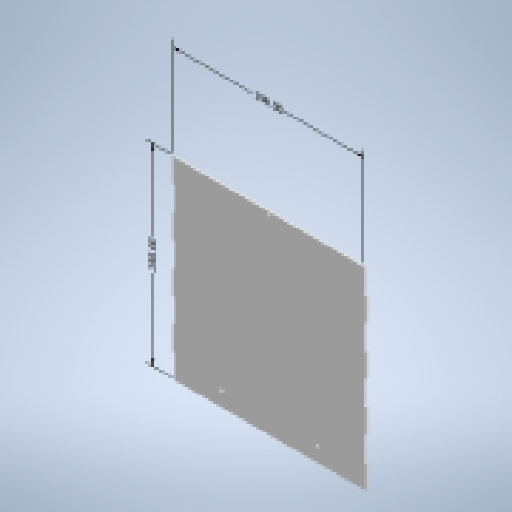
# Autodesk Inventor part: Contenedor_Pared_1
Saved by Autodesk Inventor 2024 (Build 280153000, 153)
## iProperties
Created: 2024-07-16
Part Number: Contenedor_Pared_1
Material: Genérico
Document SubType Name: Modeling
Designer: sergi
Density: 1 g/cm^3
Appearance: Valor por defecto
Author: sergi
Autodesk Inventor part; units mm, degrees
ref_plane "YZ Plane" through (0, 0, 0) normal (1, 0, 0) x (0, 1, 0)
ref_plane "XZ Plane" through (0, 0, 0) normal (0, 1, 0) x (-1, 0, 0)
ref_plane "XY Plane" through (0, 0, 0) normal (0, 0, 1) x (1, 0, 0)
sketch "Boceto1" plane through (0, 0, 0) normal (0, 0, 1) x (1, 0, 0)
  line L0 (0, 200) -> (0, 175)
  line L1 (0, 175) -> (2, 175)
  line L2 (2, 175) -> (2, 150)
  line L3 (2, 150) -> (0, 150)
  line L4 (0, 150) -> (0, 125)
  line L5 (0, 125) -> (2, 125)
  line L6 (2, 125) -> (2, 100)
  line L7 (2, 100) -> (0, 100)
  line L8 (0, 100) -> (0, 75)
  line L9 (0, 75) -> (2, 75)
  line L10 (2, 75) -> (2, 50)
  line L11 (2, 50) -> (0, 50)
  line L12 (0, 50) -> (0, 25)
  line L13 (2, 25) -> (2, 0)
  line L14 (0, 0) -> (200, 0) projected
  line L15 (0, 200) -> (200, 200) projected
  line L16 (200, 200) -> (198, 200)
  line L17 (198, 200) -> (198, 175)
  line L18 (198, 175) -> (200, 175)
  line L19 (200, 175) -> (200, 150)
  line L20 (200, 150) -> (198, 150)
  line L21 (198, 150) -> (198, 125)
  line L22 (198, 125) -> (200, 125)
  line L23 (200, 125) -> (200, 100)
  line L24 (200, 100) -> (198, 100)
  line L25 (198, 100) -> (198, 75)
  line L26 (198, 75) -> (200, 75)
  line L27 (200, 75) -> (200, 50)
  line L28 (200, 50) -> (198, 50)
  line L29 (198, 50) -> (198, 25)
  line L30 (198, 25) -> (200, 25)
  line L31 (200, 0) -> (200, 25)
  line L32 (0, 25) -> (2, 25)
  dimension "d0" = 25
  dimension "espesor" = 2
  dimension "d3" = 2
  dimension "d5" = 2
  dimension "d6" = 25
  dimension "d7" = 2
  dimension "d8" = 2
  dimension "d9" = 25
  dimension "d10" = 2
  dimension "d15" = 25
  dimension "d34" = 25
  dimension "d35" = 25
  dimension "d36" = 25
  dimension "d37" = 25
  dimension "d38" = 2
  dimension "d39" = 25
  dimension "d40" = 25
  dimension "d41" = 2
  dimension "d42" = 25
  dimension "d43" = 2
  dimension "d44" = 25
  dimension "d45" = 2
  dimension "d46" = 25
  dimension "d47" = 2
  dimension "d48" = 25
  dimension "d49" = 2
  dimension "d50" = 25
  dimension "d51" = 2
  dimension "d52" = 25
  dimension "d53" = 2
  constraints: 62 end point, 7 point on line, 4 horizontal, 4 vertical, 1 perpendicular
  measures "d0" distance of L0.start L0.end
  measures "espesor" distance of L0.end L1.end
  measures "d3" distance of L2.end L3.end
  measures "d5" distance of L5.start L5.end
  measures "d6" distance of L5.end L6.end
  measures "d7" distance of L6.end L7.end
  measures "d8" distance of L9.start L9.end
  measures "d9" distance of L9.end L10.end
  measures "d10" distance of L10.end L11.end
  measures "d15" distance of L13.start L13.end
  measures "d34" distance of L3.end L4.end
  measures "d35" distance of L1.end L2.end
  measures "d36" distance of L7.end L8.end
  measures "d37" distance of L11.end L12.end
  measures "d38" distance of L15.end L16.end
  measures "d39" distance of L16.end L17.end
  measures "d40" distance of L18.end L19.end
  measures "d41" distance of L19.end L20.end
  measures "d42" distance of L20.end L21.end
  measures "d43" distance of L21.end L22.end
  measures "d44" distance of L22.end L23.end
  measures "d45" distance of L23.end L24.end
  measures "d46" distance of L24.end L25.end
  measures "d47" distance of L25.end L26.end
  measures "d48" distance of L26.end L27.end
  measures "d49" distance of L27.end L28.end
  measures "d50" distance of L28.end L29.end
  measures "d51" distance of L29.end L30.end
  measures "d52" distance of L14.end L30.end
  measures "d53" distance of L12.end L13.start
extrude "Extrusión1" add sketch "Boceto1" against normal blind 2
sketch "Boceto2" plane through (0, 0, 0) normal (0, 0, 1) x (1, 0, 0)
  line L0 (0, 0) -> (200, 0)
  line L1 (200, 0) -> (200, 200)
  line L2 (200, 200) -> (0, 200)
  line L3 (0, 200) -> (0, 0)
  line L4 (2, 30) -> (198, 30)
  line L5 (2, 30) -> (0, 30)
  line L6 (198, 30) -> (200, 30)
  line L7 (0, 0) -> (0, 15)
  line L8 (0, 15) -> (50, 15)
  line L9 (50, 15) -> (150, 15)
  circle A0 centre (50, 15) radius 1.75
  circle A1 centre (150, 15) radius 1.75
  dimension "d54" = 15
  dimension "d55" = 50
  dimension "d56" = 100
  dimension "d57" = 3.5
  dimension "d58" = 3.5
  constraints: 20 end point, 5 point on line, 3 perpendicular, 2 centre point, 2 coincident, 2 parallel, 1 horizontal, 2 other
  measures "d54" distance of L0.start L7.end
  measures "d55" distance of L7.end L8.end
  measures "d56" distance of L8.end L9.end
  measures "d57" diameter of A0
  measures "d58" diameter of A1
extrude "Extrusión2" cut sketch "Boceto2" against normal blind 2 contours A0 L9 L8 | L8 L9 A0 | A1
sketch "Boceto4" plane through (0, 0, -2) normal (0, 0, -1) x (-1, 0, 0)
  point P0 (0, 0)
sketch "Boceto5" plane through (0, 0, -2) normal (0, 0, -1) x (-1, 0, 0)
  circle A0 centre (-150, 15) radius 1.75 projected
  circle A1 centre (-50, 15) radius 1.75 projected
  line L0 (-2, 0) -> (-2, 25) projected
  line L1 (-2, 25) -> (0, 25) projected
  line L2 (0, 25) -> (0, 50) projected
  line L3 (0, 50) -> (-2, 50) projected
  line L4 (-2, 50) -> (-2, 75) projected
  line L5 (-2, 75) -> (0, 75) projected
  line L6 (0, 75) -> (0, 100) projected
  line L7 (0, 100) -> (-2, 100) projected
  line L8 (-2, 100) -> (-2, 125) projected
  line L9 (-2, 125) -> (0, 125) projected
  line L10 (0, 125) -> (0, 150) projected
  line L11 (0, 150) -> (-2, 150) projected
  line L12 (-2, 150) -> (-2, 175) projected
  line L13 (-2, 175) -> (0, 175) projected
  line L14 (0, 175) -> (0, 200) projected
  line L15 (0, 200) -> (-198, 200) projected
  line L16 (-198, 200) -> (-198, 175) projected
  line L17 (-198, 175) -> (-200, 175) projected
  line L18 (-200, 175) -> (-200, 150) projected
  line L19 (-200, 150) -> (-198, 150) projected
  line L20 (-198, 150) -> (-198, 125) projected
  line L21 (-198, 125) -> (-200, 125) projected
  line L22 (-200, 125) -> (-200, 100) projected
  line L23 (-200, 100) -> (-198, 100) projected
  line L24 (-198, 100) -> (-198, 75) projected
  line L25 (-198, 75) -> (-200, 75) projected
  line L26 (-200, 75) -> (-200, 50) projected
  line L27 (-200, 50) -> (-198, 50) projected
  line L28 (-198, 50) -> (-198, 25) projected
  line L29 (-198, 25) -> (-200, 25) projected
  line L30 (-200, 25) -> (-200, 0) projected
  line L31 (-200, 0) -> (-2, 0) projected
  line L32 (-198, 200) -> (-198, 198)
  line L33 (-198, 200) -> (-198, 175) projected
  line L34 (-198, 198) -> (0, 198)
  point P0 (0, 0)
  dimension "d74" = 2
  constraints: 4 end point, 2 point on line, 1 perpendicular
  measures "d74" distance of L15.end L32.end
extrude "Extrusión3" cut sketch "Boceto5" against normal blind 2 contours L34 L16 L15 L14
sketch "Boceto6" plane through (0, 0, -2) normal (0, 0, -1) x (-1, 0, 0)
  line L0 (0, 198) -> (-198, 198) projected
  line L1 (-198, 198) -> (-198, 175) projected
  line L2 (-198, 175) -> (-200, 175) projected
  line L3 (-200, 175) -> (-200, 150) projected
  line L4 (-200, 150) -> (-198, 150) projected
  line L5 (-198, 150) -> (-198, 125) projected
  line L6 (-198, 125) -> (-200, 125) projected
  line L7 (-200, 125) -> (-200, 100) projected
  line L8 (-200, 100) -> (-198, 100) projected
  line L9 (-198, 100) -> (-198, 75) projected
  line L10 (-198, 75) -> (-200, 75) projected
  line L11 (-200, 75) -> (-200, 50) projected
  line L12 (-200, 50) -> (-198, 50) projected
  line L13 (-198, 50) -> (-198, 25) projected
  line L14 (-198, 25) -> (-200, 25) projected
  line L15 (-200, 25) -> (-200, 0) projected
  line L16 (-200, 0) -> (-2, 0) projected
  line L17 (-2, 0) -> (-2, 25) projected
  line L18 (-2, 25) -> (0, 25) projected
  line L19 (0, 25) -> (0, 50) projected
  line L20 (0, 50) -> (-2, 50) projected
  line L21 (-2, 50) -> (-2, 75) projected
  line L22 (-2, 75) -> (0, 75) projected
  line L23 (0, 75) -> (0, 100) projected
  line L24 (0, 100) -> (-2, 100) projected
  line L25 (-2, 100) -> (-2, 125) projected
  line L26 (-2, 125) -> (0, 125) projected
  line L27 (0, 125) -> (0, 150) projected
  line L28 (0, 150) -> (-2, 150) projected
  line L29 (-2, 150) -> (-2, 175) projected
  line L30 (-2, 175) -> (0, 175) projected
  line L31 (0, 175) -> (0, 198) projected
  circle A0 centre (-50, 15) radius 1.75 projected
  circle A1 centre (-150, 15) radius 1.75 projected
  line L32 (-99, 198) -> (-99, 195.5)
  circle A2 centre (-99, 195.5) radius 1.6
  point P0 (0, 0)
  dimension "d77" = 2.5
  dimension "d78" = 3.2
  constraints: 2 end point, 1 centre point, 1 coincident, 1 midpoint, 1 vertical
  measures "d77" distance of L32.start L32.end
  measures "d78" diameter of A2
hole "Agujero2" at (99, 195.5, -2) direction (0, 0, 1) diameter 3.2 end through all
equation "\"d0\" = Lengueta"
equation "\"d3\" = espesor"
equation "\"d5\" = espesor"
equation "\"d6\" = Lengueta"
equation "\"d7\" = espesor"
equation "\"d8\" = espesor"
equation "\"d9\" = Lengueta"
equation "\"d10\" = espesor"
equation "\"d15\" = Lengueta"
equation "\"d34\" = Lengueta"
equation "\"d35\" = Lengueta"
equation "\"d36\" = Lengueta"
equation "\"d37\" = Lengueta"
equation "\"d38\" = espesor"
equation "\"d39\" = Lengueta"
equation "\"d40\" = Lengueta"
equation "\"d41\" = espesor"
equation "\"d42\" = Lengueta"
equation "\"d43\" = espesor"
equation "\"d44\" = Lengueta"
equation "\"d45\" = espesor"
equation "\"d46\" = Lengueta"
equation "\"d47\" = espesor"
equation "\"d48\" = Lengueta"
equation "\"d49\" = espesor"
equation "\"d50\" = Lengueta"
equation "\"d51\" = espesor"
equation "\"d52\" = Lengueta"
equation "\"d53\" = espesor"
equation "\"d29\" = espesor"
equation "\"d59\" = espesor"
equation "\"d75\" = espesor"
equation "\"Lengueta\" = 25"
